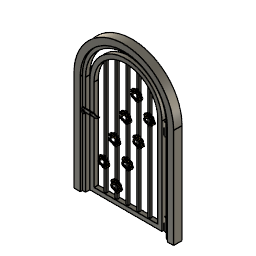
Dog+Door (Autodesk Fusion 360 archive; units mm, degrees)
design "Dog Door"
Autodesk Fusion 360 part; units mm, degrees
note: some values were not read from the file. Chosen so that the rebuilt part matches the saved one: which bodies a step acts on.
(part 1 of 3)
sketch "DJ - Baxley - Dog Door" plane through (0, 0, 0) normal (0, 1, 0) x (1, 0, 0)
  line L0 (607.7627, -514.9017) -> (801.2677, -514.9017)
  line L1 (607.7627, -512.0374) -> (758.5846, -512.0374)
  line L2 (418.6134, 33.8718) -> (522.0074, 33.8718)
  line L3 (418.6134, 36.7362) -> (541.7026, 36.7362)
  line L4 (-253.3508, 33.8718) -> (-95.7652, 33.8718)
  line L5 (-253.3508, 36.7362) -> (-129.8188, 36.7362)
  circle A0 centre (-152.9013, -288.0754) radius 7.1816
  circle A1 centre (-11.8765, -330.8233) radius 7.1816
  circle A2 centre (-21.6679, -658.9263) radius 7.1816
  circle A3 centre (53.7402, -526.3669) radius 7.1816
  circle A4 centre (-77.4932, -135.2797) radius 7.1816
  circle A5 centre (-87.2846, -473.5008) radius 7.1816
  arc A6 (65.6738, -526.867) -> (65.6738, -526.867) centre (53.7402, -526.3669) cw
  arc A7 (-9.7343, -659.4265) -> (-9.7343, -659.4265) centre (-21.6679, -658.9263) cw
  arc A8 (-140.9676, -288.5756) -> (-140.9676, -288.5756) centre (-152.9013, -288.0754) cw
  arc A9 (-65.5595, -135.7798) -> (-65.5595, -135.7798) centre (-77.4932, -135.2797) cw
  arc A10 (0.0572, -331.3234) -> (0.0572, -331.3234) centre (-11.8765, -330.8233) cw
  arc A11 (-75.351, -474.001) -> (-75.351, -474.001) centre (-87.2846, -473.5008) cw
  circle A12 centre (-61.241, -141.518) radius 7.1816
  circle A13 centre (69.9923, -532.6052) radius 7.1816
  circle A14 centre (-136.6492, -294.3137) radius 7.1816
  circle A15 centre (-71.0325, -479.7392) radius 7.1816
  circle A16 centre (4.3756, -337.0616) radius 7.1816
  circle A17 centre (-5.4158, -665.1646) radius 7.1816
  circle A18 centre (11.4514, -657.6558) radius 7.1816
  circle A19 centre (-44.3738, -134.0092) radius 7.1816
  circle A20 centre (21.2429, -329.5528) radius 7.1816
  circle A21 centre (-119.7819, -286.8049) radius 7.1816
  circle A22 centre (86.8596, -525.0964) radius 7.1816
  circle A23 centre (-54.1652, -472.2303) radius 7.1816
  arc A24 (-129.4885, -293.765) -> (-129.4885, -293.765) centre (-119.7819, -286.8049) cw
  arc A25 (1.7448, -664.6159) -> (1.7448, -664.6159) centre (11.4514, -657.6558) cw
  arc A26 (-54.0804, -140.9693) -> (-54.0804, -140.9693) centre (-44.3738, -134.0092) cw
  arc A27 (77.1529, -532.0565) -> (77.1529, -532.0565) centre (86.8596, -525.0964) cw
  arc A28 (-63.8719, -479.1905) -> (-63.8719, -479.1905) centre (-54.1652, -472.2303) cw
  arc A29 (11.5363, -336.5129) -> (11.5363, -336.5129) centre (21.2429, -329.5528) cw
  circle A30 centre (27.4799, -313.3013) radius 7.1825
  circle A31 centre (-47.9282, -455.9788) radius 7.1825
  circle A32 centre (-38.1368, -117.7577) radius 7.1825
  circle A33 centre (17.6884, -641.4043) radius 7.1825
  circle A34 centre (-113.5449, -270.5534) radius 7.1825
  circle A35 centre (93.0966, -508.8449) radius 7.1825
  arc A36 (-123.6388, -263.5828) -> (-125.432, -269.8418) centre (-116.4072, -269.0411) ccw
  arc A37 (61.7026, -517.6651) -> (60.8566, -516.7375) centre (51.8781, -525.7767) ccw
  arc A38 (81.2094, -508.1333) -> (81.353, -509.5872) centre (62.2283, -510.7421) cw
  arc A39 (-125.432, -269.8418) -> (-125.2884, -271.2957) centre (-144.4132, -272.4506) cw
  arc A40 (7.5945, -634.4337) -> (5.8013, -640.6927) centre (14.8261, -639.892) ccw
  arc A41 (-139.7053, -250.77) -> (-138.4238, -249.5216) centre (-127.7264, -261.7846) cw
  arc A42 (-75.2386, -123.1969) -> (-77.5786, -122.844) centre (-74.3062, -109.0815) cw
  arc A43 (54.9363, -493.7824) -> (58.1264, -493.5058) centre (54.4348, -469.4584) ccw
  arc A44 (-95.1258, -450.308) -> (-86.0885, -440.9163) centre (-84.8968, -451.1071) cw
  arc A45 (5.8013, -640.6927) -> (5.9449, -642.1466) centre (-13.1798, -643.3015) cw
  arc A46 (-59.8154, -455.2673) -> (-59.6718, -456.7212) centre (-78.7965, -457.8761) cw
  arc A47 (-50.0239, -117.0461) -> (-49.8803, -118.5) centre (-69.005, -119.6549) cw
  arc A48 (-72.8072, -434.947) -> (-58.0221, -449.0083) centre (-66.1625, -442.764) cw
  arc A49 (-59.6718, -456.7212) -> (-79.3222, -464.799) centre (-70.9412, -457.2469) cw
  arc A50 (45.899, -503.1741) -> (54.9363, -493.7824) centre (56.128, -503.9731) cw
  arc A51 (-152.9867, -275.6397) -> (-160.7425, -264.8826) centre (-150.5091, -265.6789) cw
  arc A52 (-150.6468, -275.9926) -> (-152.9867, -275.6397) centre (-149.7143, -261.8772) cw
  arc A53 (55.9947, -514.2841) -> (53.6548, -513.9312) centre (56.9271, -500.1687) cw
  arc A54 (-70.3768, -125.6503) -> (-75.2386, -123.1969) centre (-76.6948, -132.1266) ccw
  arc A55 (60.8566, -516.7375) -> (55.9947, -514.2841) centre (54.5386, -523.2138) ccw
  arc A56 (-64.2972, -97.9742) -> (-63.0157, -96.7259) centre (-52.3183, -108.9889) cw
  arc A57 (-73.107, -102.4186) -> (-64.2972, -97.9742) centre (-75.763, -86.2002) ccw
  arc A58 (-48.2307, -110.7871) -> (-50.0239, -117.0461) centre (-40.9991, -116.2454) ccw
  arc A59 (-77.5786, -122.844) -> (-85.3344, -112.0869) centre (-75.1009, -112.8832) cw
  arc A60 (-9.622, -318.7405) -> (-11.9619, -318.3876) centre (-8.6895, -304.6251) cw
  arc A61 (66.9361, -489.0615) -> (68.2176, -487.8131) centre (78.915, -500.0761) cw
  arc A62 (-7.4903, -297.9622) -> (1.3195, -293.5179) centre (-10.1463, -281.7438) ccw
  arc A63 (-3.9141, -322.1215) -> (-4.7601, -321.1939) centre (-13.7386, -330.2331) ccw
  arc A64 (-85.3344, -112.0869) -> (-76.297, -102.6952) centre (-75.1054, -112.8859) cw
  arc A65 (15.5928, -312.5897) -> (15.7364, -314.0436) centre (-3.3884, -315.1985) cw
  arc A66 (53.6548, -513.9312) -> (45.899, -503.1741) centre (56.1324, -503.9704) cw
  arc A67 (-82.8984, -440.6398) -> (-74.0887, -436.1954) centre (-85.5544, -424.4213) ccw
  arc A68 (58.1264, -493.5058) -> (66.9361, -489.0615) centre (55.4703, -477.2874) ccw
  arc A69 (-58.0221, -449.0083) -> (-59.8154, -455.2673) centre (-50.7905, -454.4665) ccw
  arc A70 (2.6009, -292.2695) -> (17.386, -306.3307) centre (9.2456, -300.0864) cw
  arc A71 (1.3195, -293.5179) -> (2.6009, -292.2695) centre (13.2983, -304.5325) cw
  arc A72 (-145.7849, -278.446) -> (-150.6468, -275.9926) centre (-152.1029, -284.9223) ccw
  arc A73 (-138.4238, -249.5216) -> (-123.6388, -263.5828) centre (-131.7791, -257.3385) cw
  arc A74 (-144.9389, -279.3736) -> (-145.7849, -278.446) centre (-154.7633, -287.4852) ccw
  arc A75 (-160.7425, -264.8826) -> (-151.7051, -255.4909) centre (-150.5135, -265.6816) cw
  arc A76 (-49.8803, -118.5) -> (-69.5307, -126.5778) centre (-61.1497, -119.0257) cw
  arc A77 (-69.5307, -126.5778) -> (-70.3768, -125.6503) centre (-79.3552, -134.6895) ccw
  arc A78 (-74.0887, -436.1954) -> (-72.8072, -434.947) centre (-62.1098, -447.2101) cw
  arc A79 (-7.1905, -620.3725) -> (7.5945, -634.4337) centre (-0.5458, -628.1894) cw
  arc A80 (-86.0885, -440.9163) -> (-82.8984, -440.6398) centre (-86.59, -416.5924) ccw
  arc A81 (-85.0301, -461.4181) -> (-87.37, -461.0652) centre (-84.0977, -447.3027) cw
  arc A82 (-4.7601, -321.1939) -> (-9.622, -318.7405) centre (-11.0781, -327.6702) ccw
  arc A83 (-87.37, -461.0652) -> (-95.1258, -450.308) centre (-84.8924, -451.1043) cw
  arc A84 (81.353, -509.5872) -> (61.7026, -517.6651) centre (70.0836, -510.1129) cw
  arc A85 (-79.3222, -464.799) -> (-80.1682, -463.8715) centre (-89.1467, -472.9106) ccw
  arc A86 (-125.2884, -271.2957) -> (-144.9389, -279.3736) centre (-136.5578, -271.8214) cw
  arc A87 (-76.297, -102.6952) -> (-73.107, -102.4186) centre (-76.7985, -78.3712) ccw
  arc A88 (83.0027, -501.8743) -> (81.2094, -508.1333) centre (90.2342, -507.3326) ccw
  arc A89 (-10.6804, -298.2388) -> (-7.4903, -297.9622) centre (-11.1819, -273.9148) ccw
  arc A90 (-151.7051, -255.4909) -> (-148.5151, -255.2144) centre (-152.2066, -231.1669) ccw
  arc A91 (-63.0157, -96.7259) -> (-48.2307, -110.7871) centre (-56.371, -104.5428) cw
  arc A92 (-13.7055, -650.2245) -> (-14.5516, -649.2969) centre (-23.53, -658.3361) ccw
  arc A93 (-80.1682, -463.8715) -> (-85.0301, -461.4181) centre (-86.4862, -470.3477) ccw
  arc A94 (-17.2817, -626.0653) -> (-8.472, -621.6209) centre (-19.9378, -609.8468) ccw
  arc A95 (-19.4134, -646.8435) -> (-21.7533, -646.4906) centre (-18.481, -632.7281) cw
  arc A96 (-11.9619, -318.3876) -> (-19.7177, -307.6305) centre (-9.4843, -308.4268) cw
  arc A97 (68.2176, -487.8131) -> (83.0027, -501.8743) centre (74.8623, -495.63) cw
  arc A98 (-148.5151, -255.2144) -> (-139.7053, -250.77) centre (-151.1711, -238.9959) ccw
  arc A99 (-29.5091, -635.7335) -> (-20.4718, -626.3418) centre (-19.2801, -636.5325) cw
  arc A100 (5.9449, -642.1466) -> (-13.7055, -650.2245) centre (-5.3245, -642.6723) cw
  arc A101 (15.7364, -314.0436) -> (-3.9141, -322.1215) centre (4.4669, -314.5693) cw
  arc A102 (-14.5516, -649.2969) -> (-19.4134, -646.8435) centre (-20.8696, -655.7732) ccw
  arc A103 (-8.472, -621.6209) -> (-7.1905, -620.3725) centre (3.5069, -632.6355) cw
  arc A104 (17.386, -306.3307) -> (15.5928, -312.5897) centre (24.6176, -311.789) ccw
  arc A105 (-19.7177, -307.6305) -> (-10.6804, -298.2388) centre (-9.4887, -308.4295) cw
  arc A106 (-20.4718, -626.3418) -> (-17.2817, -626.0653) centre (-20.9733, -602.0178) ccw
  arc A107 (-21.7533, -646.4906) -> (-29.5091, -635.7335) centre (-19.2757, -636.5298) cw
  arc A108 (-2.0837, -290.1836) -> (-0.5075, -288.6612) centre (13.2983, -304.5325) cw
  arc A109 (-77.4918, -432.8611) -> (-75.9156, -431.3388) centre (-62.1098, -447.2101) cw
  arc A110 (-10.9728, -293.4803) -> (-8.2372, -293.2586) centre (-11.1819, -273.9148) ccw
  arc A111 (-75.9156, -431.3388) -> (-51.2415, -444.5025) centre (-66.1625, -442.764) cw
  arc A112 (-34.2572, -635.3633) -> (-20.7643, -621.5833) centre (-19.2801, -636.5325) cw
  arc A113 (-6.6815, -341.5785) -> (-18.1828, -320.68) centre (-11.8765, -330.8234) cw
  arc A114 (-11.8752, -618.2866) -> (-10.2989, -616.7642) centre (3.5069, -632.6355) cw
  arc A115 (14.3752, -629.9279) -> (22.2071, -652.4617) centre (17.6884, -641.4043) cw
  arc A116 (-16.473, -669.6815) -> (-27.9743, -648.783) centre (-21.668, -658.9264) cw
  arc A117 (-93.591, -463.3575) -> (-99.8739, -449.9379) centre (-84.8924, -451.1043) cw
  arc A118 (81.5082, -535.7746) -> (58.9352, -537.1221) centre (69.9923, -532.6052) cw
  arc A119 (63.533, -485.7272) -> (65.1092, -484.2048) centre (78.915, -500.0761) cw
  arc A120 (47.4338, -516.2236) -> (41.1509, -502.8039) centre (56.1324, -503.9704) cw
  arc A121 (57.3795, -488.8022) -> (63.533, -485.7272) centre (55.4703, -477.2874) ccw
  arc A122 (41.1509, -502.8039) -> (54.6438, -489.0239) centre (56.128, -503.9731) cw
  arc A123 (89.7833, -497.3685) -> (97.6152, -519.9023) centre (93.0966, -508.8449) cw
  arc A124 (54.6438, -489.0239) -> (57.3795, -488.8022) centre (54.4348, -469.4584) ccw
  arc A125 (65.1092, -484.2048) -> (89.7833, -497.3685) centre (74.8623, -495.63) cw
  arc A126 (-66.1242, -93.1176) -> (-41.45, -106.2813) centre (-56.371, -104.5428) cw
  arc A127 (-86.3809, -436.1579) -> (-83.6453, -435.9362) centre (-86.59, -416.5924) ccw
  arc A128 (-143.1085, -247.4357) -> (-141.5323, -245.9133) centre (-127.7264, -261.7846) cw
  arc A129 (-159.2076, -277.9321) -> (-165.4906, -264.5124) centre (-150.5091, -265.6789) cw
  arc A130 (-49.7251, -144.6874) -> (-72.2982, -146.0349) centre (-61.241, -141.518) cw
  arc A131 (-141.5323, -245.9133) -> (-116.8581, -259.077) centre (-131.7791, -257.3385) cw
  arc A132 (-109.0263, -281.6108) -> (-125.1332, -297.4832) centre (-119.7819, -286.8049) cw
  arc A133 (-83.7995, -125.1364) -> (-90.0824, -111.7167) centre (-75.1009, -112.8832) cw
  arc A134 (-90.0824, -111.7167) -> (-76.5895, -97.9367) centre (-75.1054, -112.8859) cw
  arc A135 (-67.7004, -94.64) -> (-66.1242, -93.1176) centre (-52.3183, -108.9889) cw
  arc A136 (-165.4906, -264.5124) -> (-151.9976, -250.7324) centre (-150.5135, -265.6816) cw
  arc A137 (-76.5895, -97.9367) -> (-73.8539, -97.715) centre (-76.7985, -78.3712) ccw
  arc A138 (-125.1332, -297.4832) -> (-147.7063, -298.8306) centre (-136.6492, -294.3137) cw
  arc A139 (-82.0896, -484.2561) -> (-93.591, -463.3575) centre (-87.2847, -473.501) cw
  arc A140 (-116.8581, -259.077) -> (-109.0263, -281.6108) centre (-113.5449, -270.5534) cw
  arc A141 (-151.9976, -250.7324) -> (-149.262, -250.5107) centre (-152.2066, -231.1669) ccw
  arc A142 (-73.8539, -97.715) -> (-67.7004, -94.64) centre (-75.763, -86.2002) ccw
  arc A143 (-33.6181, -128.815) -> (-49.7251, -144.6874) centre (-44.3738, -134.0092) cw
  arc A144 (-72.2982, -146.0349) -> (-83.7995, -125.1364) centre (-77.4932, -135.2798) cw
  arc A145 (-147.7063, -298.8306) -> (-159.2076, -277.9321) centre (-152.9013, -288.0755) cw
  arc A146 (-149.262, -250.5107) -> (-143.1085, -247.4357) centre (-151.1711, -238.9959) ccw
  arc A147 (-41.45, -106.2813) -> (-33.6181, -128.815) centre (-38.1368, -117.7577) cw
  arc A148 (-99.8739, -449.9379) -> (-86.3809, -436.1579) centre (-84.8968, -451.1071) cw
  arc A149 (-43.4096, -467.0362) -> (-59.5166, -482.9086) centre (-54.1652, -472.2303) cw
  arc A150 (-8.2372, -293.2586) -> (-2.0837, -290.1836) centre (-10.1463, -281.7438) ccw
  arc A151 (-18.0287, -621.3616) -> (-11.8752, -618.2866) centre (-19.9378, -609.8468) ccw
  arc A152 (31.9985, -324.3586) -> (15.8916, -340.231) centre (21.2429, -329.5528) cw
  arc A153 (15.8916, -340.231) -> (-6.6815, -341.5785) centre (4.3756, -337.0616) cw
  arc A154 (97.6152, -519.9023) -> (81.5082, -535.7746) centre (86.8596, -525.0964) cw
  arc A155 (-18.1828, -320.68) -> (-24.4658, -307.2603) centre (-9.4843, -308.4268) cw
  arc A156 (-59.5166, -482.9086) -> (-82.0896, -484.2561) centre (-71.0325, -479.7392) cw
  arc A157 (-24.4658, -307.2603) -> (-10.9728, -293.4803) centre (-9.4887, -308.4295) cw
  arc A158 (-27.9743, -648.783) -> (-34.2572, -635.3633) centre (-19.2757, -636.5298) cw
  arc A159 (-83.6453, -435.9362) -> (-77.4918, -432.8611) centre (-85.5544, -424.4213) ccw
  arc A160 (-20.7643, -621.5833) -> (-18.0287, -621.3616) centre (-20.9733, -602.0178) ccw
  arc A161 (-0.5075, -288.6612) -> (24.1667, -301.8249) centre (9.2456, -300.0864) cw
  arc A162 (-51.2415, -444.5025) -> (-43.4096, -467.0362) centre (-47.9282, -455.9788) cw
  arc A163 (-10.2989, -616.7642) -> (14.3752, -629.9279) centre (-0.5458, -628.1894) cw
  arc A164 (22.2071, -652.4617) -> (6.1001, -668.3341) centre (11.4514, -657.6558) cw
  arc A165 (6.1001, -668.3341) -> (-16.473, -669.6815) centre (-5.4158, -665.1646) cw
  arc A166 (58.9352, -537.1221) -> (47.4338, -516.2236) centre (53.7401, -526.367) cw
  arc A167 (24.1667, -301.8249) -> (31.9985, -324.3586) centre (27.4799, -313.3013) cw
  line L6 (-608.6223, -1298.6439) -> (1173.7004, -1298.6439)
  line L7 (1173.7004, -1298.6439) -> (1173.7004, 250.0202)
  line L8 (1173.7004, 250.0202) -> (-608.6223, 250.0202)
  line L9 (-608.6223, 250.0202) -> (-608.6223, -1298.6439)
  line L10 (-241.1509, 0) -> (-241.1509, -411.8539)
  line L11 (241.4491, -596.9) -> (241.4491, 0)
  line L12 (-241.1509, -439.1647) -> (-241.1509, -596.9)
  arc A168 (-241.1509, -596.9) -> (241.4491, -596.9) centre (0.1491, -596.9) ccw
  line L13 (-215.7509, -439.1647) -> (-215.7509, -596.9)
  line L14 (-215.7509, -25.4) -> (-215.7509, -420.1147)
  line L15 (216.0491, -25.4) -> (-215.7509, -25.4)
  line L16 (216.0491, -596.9) -> (216.0491, -25.4)
  arc A169 (-215.7509, -596.9) -> (216.0491, -596.9) centre (0.1491, -596.9) ccw
  line L17 (-190.3509, -50.8) -> (-190.3509, -420.1147)
  arc A170 (-190.3509, -596.9) -> (190.6491, -596.9) centre (0.1491, -596.9) ccw
  line L18 (190.6491, -596.9) -> (190.6491, -50.8)
  line L19 (-190.3509, -439.1647) -> (-190.3509, -596.9)
  line L20 (190.6491, -50.8) -> (-190.3509, -50.8)
  circle A171 centre (-203.0509, -429.6397) radius 6.35
  line L21 (-253.8509, -411.8539) -> (-241.1509, -411.8539)
  line L22 (-241.1509, -411.8539) -> (-241.1509, -428.0522)
  line L23 (-253.8509, -428.0522) -> (-253.8509, -411.8539)
  line L24 (-241.1509, -428.0522) -> (-253.8509, -428.0522)
  line L25 (-181.8374, -420.1147) -> (-241.1509, -420.1147)
  line L26 (-255.4225, -439.1647) -> (-186.7302, -439.1647)
  arc A172 (-184.4429, -438.341) -> (-152.1305, -436.5446) centre (-167.2009, -456.9736) cw
  line L27 (-253.8509, -420.1147) -> (-255.4225, -420.1147)
  arc A173 (-152.1305, -436.5446) -> (-151.004, -435.1368) centre (-151.705, -435.7305) ccw
  arc A174 (-151.004, -435.1368) -> (-181.8374, -420.1147) centre (-180.7971, -457.1339) ccw
  arc A175 (-255.4225, -420.1147) -> (-255.4225, -439.1647) centre (-230.008, -429.6397) ccw
  arc A176 (-186.7302, -439.1647) -> (-184.4429, -438.341) centre (-186.7379, -435.5556) ccw
  line L28 (222.3991, -25.4) -> (235.0991, -25.4)
  line L29 (222.3991, -101.6) -> (222.3991, -25.4)
  line L30 (235.0991, -25.4) -> (235.0991, -101.6)
  line L31 (235.0991, -101.6) -> (222.3991, -101.6)
  line L32 (222.3991, -63.5) -> (235.0991, -63.5)
  line L33 (222.3991, -25.4) -> (216.0491, -25.4)
  line L34 (222.3991, -63.5) -> (222.3991, -25.4)
  line L35 (216.0491, -63.5) -> (222.3991, -63.5)
  line L36 (216.0491, -25.4) -> (216.0491, -63.5)
  line L37 (235.0991, -101.6) -> (241.4491, -101.6)
  line L38 (241.4491, -101.6) -> (241.4491, -63.5)
  line L39 (241.4491, -63.5) -> (235.0991, -63.5)
  line L40 (235.0991, -63.5) -> (235.0991, -101.6)
  line L41 (222.3991, -594.9254) -> (222.3991, -518.7254)
  line L42 (235.0991, -518.7254) -> (235.0991, -594.9254)
  line L43 (222.3991, -518.7254) -> (235.0991, -518.7254)
  line L44 (235.0991, -594.9254) -> (222.3991, -594.9254)
  line L45 (222.3991, -556.8254) -> (235.0991, -556.8254)
  line L46 (222.3991, -556.8254) -> (222.3991, -518.7254)
  line L47 (216.0491, -518.7254) -> (216.0491, -556.8254)
  line L48 (216.0491, -556.8254) -> (222.3991, -556.8254)
  line L49 (222.3991, -518.7254) -> (216.0491, -518.7254)
  line L50 (235.0991, -594.9254) -> (241.4491, -594.9254)
  line L51 (241.4491, -556.8254) -> (235.0991, -556.8254)
  line L52 (241.4491, -594.9254) -> (241.4491, -556.8254)
  line L53 (235.0991, -556.8254) -> (235.0991, -594.9254)
  line L54 (6.4991, -50.8) -> (6.4991, -285.3177)
  line L55 (6.4991, -290.2014) -> (6.4991, -325.6665)
  line L56 (6.4991, -330.2011) -> (6.4991, -343.9221)
  line L57 (6.4991, -348.8155) -> (6.4991, -614.9219)
  line L58 (6.4991, -620.7312) -> (6.4991, -636.3213)
  line L59 (6.4991, -652.4548) -> (6.4991, -662.8568)
  line L60 (6.4991, -668.5249) -> (6.4991, -787.2941)
  line L61 (-6.2009, -50.8) -> (-6.2009, -292.7287)
  line L62 (-6.2009, -297.6977) -> (-6.2009, -320.3138)
  line L63 (-6.2009, -326.4229) -> (-6.2009, -335.2236)
  line L64 (-6.2009, -342.6114) -> (-6.2009, -614.2725)
  line L65 (-6.2009, -619.6292) -> (-6.2009, -653.9199)
  line L66 (-6.2009, -658.0261) -> (-6.2009, -672.3032)
  line L67 (-6.2009, -677.083) -> (-6.2009, -787.2941)
  line L68 (-59.1175, -50.8) -> (-59.1175, -89.7741)
  line L69 (-59.1175, -94.6578) -> (-59.1175, -130.1228)
  line L70 (-59.1175, -134.6575) -> (-59.1175, -148.3785)
  line L71 (-59.1175, -153.2719) -> (-59.1175, -429.4964)
  line L72 (-59.1175, -435.3057) -> (-59.1175, -450.8958)
  line L73 (-59.1175, -467.0293) -> (-59.1175, -477.4313)
  line L74 (-59.1175, -483.0994) -> (-59.1175, -777.9462)
  line L75 (-71.8175, -50.8) -> (-71.8175, -97.1851)
  line L76 (-71.8175, -102.1541) -> (-71.8175, -124.5061)
  line L77 (-71.8175, -130.8793) -> (-71.8175, -139.68)
  line L78 (-71.8175, -147.0678) -> (-71.8175, -428.8471)
  line L79 (-71.8175, -434.2038) -> (-71.8175, -468.4945)
  line L80 (-71.8175, -472.6006) -> (-71.8175, -486.8778)
  line L81 (-71.8175, -491.6575) -> (-71.8175, -773.2832)
  line L82 (72.1158, -50.8) -> (72.1158, -480.8613)
  line L83 (72.1158, -485.745) -> (72.1158, -521.2101)
  line L84 (72.1158, -525.7447) -> (72.1158, -539.4657)
  line L85 (72.1158, -544.3591) -> (72.1158, -773.2832)
  line L86 (59.4158, -50.8) -> (59.4158, -488.2723)
  line L87 (59.4158, -493.2413) -> (59.4158, -515.8574)
  line L88 (59.4158, -521.9665) -> (59.4158, -530.7672)
  line L89 (59.4158, -538.155) -> (59.4158, -777.9462)
  line L90 (137.7325, -50.8) -> (137.7325, -728.6614)
  line L91 (125.0325, -50.8) -> (125.0325, -740.7555)
  line L92 (-124.7342, -50.8) -> (-124.7342, -244.071)
  line L93 (-124.7342, -249.8803) -> (-124.7342, -265.4704)
  line L94 (-124.7342, -281.6039) -> (-124.7342, -292.0059)
  line L95 (-124.7342, -297.674) -> (-124.7342, -740.7555)
  line L96 (-137.4342, -50.8) -> (-137.4342, -243.4216)
  line L97 (-137.4342, -248.7783) -> (-137.4342, -283.069)
  line L98 (-137.4342, -287.1751) -> (-137.4342, -301.4523)
  line L99 (-137.4342, -285.9415) -> (-137.4342, -728.6614)
  line L100 (460.8307, -38.1) -> (486.2307, -38.1)
  line L101 (460.8307, -12.7) -> (460.8307, -38.1)
  line L102 (486.2307, -12.7) -> (460.8307, -12.7)
  line L103 (486.2307, -38.1) -> (486.2307, -12.7)
  line L104 (943.4307, -12.7) -> (511.6307, -12.7)
  line L105 (943.4307, -38.1) -> (943.4307, -12.7)
  line L106 (511.6307, -12.7) -> (511.6307, -38.1)
  line L107 (511.6307, -38.1) -> (943.4307, -38.1)
  line L108 (517.9807, -12.7) -> (517.9807, -9.356)
  line L109 (530.6807, -12.7) -> (530.6807, -9.356)
  line L110 (473.5307, -12.7) -> (473.5307, -9.356)
  line L111 (486.2307, -12.7) -> (486.2307, -9.356)
  line L112 (540.5255, -9.356) -> (469.714, -9.356)
  line L113 (469.714, -6.181) -> (540.5255, -6.181)
  line L114 (540.5255, -6.181) -> (540.5255, -9.356)
  line L115 (469.714, -9.356) -> (469.714, -6.181)
  line L116 (473.5307, -6.181) -> (473.5307, -2.837)
  line L117 (486.2307, -6.181) -> (486.2307, -2.837)
  line L118 (473.5307, -2.837) -> (486.2307, -2.837)
  line L119 (994.2307, -38.1) -> (994.2307, -12.7)
  line L120 (994.2307, -12.7) -> (968.8307, -12.7)
  line L121 (968.8307, -12.7) -> (968.8307, -38.1)
  line L122 (968.8307, -38.1) -> (994.2307, -38.1)
  line L123 (962.4807, -12.7) -> (962.4807, -38.1)
  line L124 (968.8307, -38.1) -> (968.8307, -12.7)
  line L125 (968.8307, -12.7) -> (962.4807, -12.7)
  line L126 (962.4807, -38.1) -> (968.8307, -38.1)
  line L127 (949.7807, -38.1) -> (949.7807, -12.7)
  line L128 (943.4307, -38.1) -> (949.7807, -38.1)
  line L129 (949.7807, -12.7) -> (943.4307, -12.7)
  line L130 (943.4307, -12.7) -> (943.4307, -38.1)
  circle A177 centre (956.1307, -12.7) radius 6.35
  arc A178 (260.4991, -596.9) -> (-260.2009, -596.9) centre (0.1491, -596.9) cw
  line L131 (260.4991, 0) -> (260.4991, -596.9)
  line L132 (-260.2009, -596.9) -> (-260.2009, 0)
  line L133 (460.8307, -12.7) -> (467.1807, -12.7)
  line L134 (467.1807, -7.9375) -> (429.0807, -7.9375)
  line L135 (467.1807, -12.7) -> (467.1807, -7.9375)
  line L136 (429.0807, -7.9375) -> (429.0807, -12.7)
  line L137 (1026.0501, -7.9375) -> (1026.0501, -12.7)
  line L138 (987.9501, -12.7) -> (987.9501, -7.9375)
  line L139 (987.9501, -7.9375) -> (1026.0501, -7.9375)
  line L140 (467.1807, -189.5481) -> (987.9501, -189.5481)
  line L141 (-298.3009, -596.9) -> (-298.3009, 0)
  arc A179 (298.5991, -596.9) -> (-298.3009, -596.9) centre (0.1491, -596.9) cw
  line L142 (298.5991, 0) -> (298.5991, -596.9)
  circle A180 centre (654.6615, -728.3062) radius 28.7265
  arc A181 (702.3961, -730.3068) -> (702.3961, -730.3068) centre (654.6615, -728.3062) cw
  circle A182 centre (719.6699, -753.2596) radius 28.7265
  circle A183 centre (787.139, -723.2242) radius 28.7265
  arc A184 (748.3124, -751.0647) -> (748.3124, -751.0647) centre (787.139, -723.2242) cw
  circle A185 centre (812.087, -658.2181) radius 28.7301
  arc A186 (707.4452, -579.0845) -> (712.5712, -574.091) centre (755.3608, -623.1431) cw
  arc A187 (771.7114, -630.3359) -> (764.5384, -655.372) centre (800.6377, -652.169) ccw
  arc A188 (659.446, -597.9682) -> (672.2062, -596.862) centre (657.44, -500.6724) ccw
  arc A189 (654.3198, -678.5635) -> (623.2966, -635.535) centre (664.2303, -638.7201) cw
  arc A190 (623.2966, -635.535) -> (659.446, -597.9682) centre (664.2126, -638.731) cw
  arc A191 (663.6795, -679.9752) -> (654.3198, -678.5635) centre (667.4092, -623.5135) cw
  arc A192 (712.5712, -574.091) -> (771.7114, -630.3359) centre (739.15, -605.3587) cw
  arc A193 (672.2062, -596.862) -> (707.4452, -579.0845) centre (661.5821, -531.9882) ccw
  arc A194 (764.5384, -655.372) -> (765.1128, -661.1875) centre (688.6139, -665.8071) cw
  arc A195 (765.1128, -661.1875) -> (686.5111, -693.4989) centre (720.0352, -663.2904) cw
  arc A196 (683.1269, -689.7887) -> (663.6795, -679.9752) centre (657.855, -715.6938) ccw
  arc A197 (686.5111, -693.4989) -> (683.1269, -689.7887) centre (647.2131, -725.9453) ccw
  arc A198 (675.4413, -771.3271) -> (629.436, -687.7329) centre (654.6613, -728.3068) cw
  arc A199 (669.2186, -578.0475) -> (693.8326, -565.7473) centre (661.5821, -531.9882) ccw
  arc A200 (629.436, -687.7329) -> (604.3043, -634.0543) centre (664.2303, -638.7201) cw
  arc A201 (693.8326, -565.7473) -> (700.1374, -559.6579) centre (755.3608, -623.1431) cw
  arc A202 (604.3043, -634.0543) -> (658.2761, -578.9344) centre (664.2126, -638.731) cw
  arc A203 (658.2761, -578.9344) -> (669.2186, -578.0475) centre (657.44, -500.6724) ccw
  arc A204 (765.7337, -765.9373) -> (675.4413, -771.3271) centre (719.6699, -753.2596) cw
  arc A205 (830.1615, -702.4477) -> (765.7337, -765.9373) centre (787.139, -723.2242) cw
  arc A206 (798.834, -612.3128) -> (830.1615, -702.4477) centre (812.087, -658.2181) cw
  arc A207 (700.1374, -559.6579) -> (798.834, -612.3128) centre (739.15, -605.3587) cw
  arc A208 (884.2022, -372.9919) -> (903.2522, -353.9419) centre (903.2522, -372.9919) cw
  line L143 (541.3022, -372.9919) -> (884.2022, -372.9919)
  arc A209 (560.3522, -220.5919) -> (541.3022, -239.6419) centre (541.3022, -220.5919) cw
  line L144 (903.2522, -353.9419) -> (903.2522, -220.5919)
  line L145 (903.2522, -220.5919) -> (560.3522, -220.5919)
  line L146 (541.3022, -239.6419) -> (541.3022, -372.9919)
  line L147 (912.7772, -211.0669) -> (912.7772, -382.5169)
  line L148 (912.7772, -211.0669) -> (531.7772, -211.0669)
  line L149 (531.7772, -211.0669) -> (531.7772, -382.5169)
  line L150 (531.7772, -382.5169) -> (912.7772, -382.5169)
  line L151 (320.6208, 0) -> (-320.6208, 0)
  line L152 (403.6807, -26.9875) -> (403.6807, -115.8875)
  line L153 (365.5807, -115.8875) -> (365.5807, -26.9875)
  line L154 (365.5807, -26.9875) -> (403.6807, -26.9875)
  line L155 (1089.5501, -115.8875) -> (1089.5501, -26.9875)
  line L156 (403.6807, -115.8875) -> (365.5807, -115.8875)
  line L157 (1051.4501, -115.8875) -> (1089.5501, -115.8875)
  line L158 (1051.4501, -26.9875) -> (1051.4501, -115.8875)
  line L159 (1089.5501, -26.9875) -> (1051.4501, -26.9875)
  line L160 (1089.5501, -26.9875) -> (1051.4501, -115.8875)
  line L161 (365.5807, -26.9875) -> (403.6807, -115.8875)
  line L162 (1051.4501, -26.9875) -> (1089.5501, -115.8875)
  line L163 (403.6807, -26.9875) -> (365.5807, -115.8875)
  line L164 (1013.3501, -115.8875) -> (1013.3501, -26.9875)
  line L165 (1106.7139, -115.8875) -> (1013.3501, -115.8875)
  line L166 (1013.3501, -26.9875) -> (1106.7139, -26.9875)
  line L167 (1013.3501, -26.9875) -> (1051.4501, -115.8875)
  line L168 (1051.4501, -26.9875) -> (1013.3501, -115.8875)
  line L169 (1051.4501, -115.8875) -> (1051.4501, -26.9875)
  line L170 (348.4169, -115.8875) -> (441.7807, -115.8875)
  line L171 (441.7807, -26.9875) -> (348.4169, -26.9875)
  line L172 (441.7807, -115.8875) -> (441.7807, -26.9875)
  line L173 (441.7807, -26.9875) -> (403.6807, -115.8875)
  line L174 (403.6807, -26.9875) -> (441.7807, -115.8875)
  line L175 (403.6807, -115.8875) -> (403.6807, -26.9875)
  line L176 (994.3001, -149.225) -> (1013.3501, -12.7)
  line L177 (994.3001, -12.7) -> (1013.3501, -149.225)
  line L178 (1013.3501, -149.225) -> (994.3001, -149.225)
  line L179 (994.3001, -149.225) -> (994.3001, -12.7)
  line L180 (994.3001, -12.7) -> (1013.3501, -12.7)
  line L181 (1013.3501, -12.7) -> (1013.3501, -149.225)
  line L182 (460.8307, -149.225) -> (441.7807, -12.7)
  line L183 (460.8307, -12.7) -> (441.7807, -149.225)
  line L184 (460.8307, -12.7) -> (441.7807, -12.7)
  line L185 (460.8307, -149.225) -> (460.8307, -12.7)
  line L186 (441.7807, -12.7) -> (441.7807, -149.225)
  line L187 (441.7807, -149.225) -> (460.8307, -149.225)
  line L188 (352.4174, -149.225) -> (441.7807, -130.175)
  line L189 (441.7807, -149.225) -> (352.4174, -130.175)
  line L190 (441.7807, -149.225) -> (441.7807, -130.175)
  line L191 (352.4174, -130.175) -> (352.4174, -149.225)
  line L192 (441.7807, -130.175) -> (352.4174, -130.175)
  line L193 (352.4174, -149.225) -> (441.7807, -149.225)
  line L194 (1102.7134, -149.225) -> (1013.3501, -130.175)
  line L195 (1013.3501, -149.225) -> (1102.7134, -130.175)
  line L196 (1102.7134, -130.175) -> (1102.7134, -149.225)
  line L197 (1013.3501, -130.175) -> (1102.7134, -130.175)
  line L198 (1102.7134, -149.225) -> (1013.3501, -149.225)
  line L199 (1013.3501, -149.225) -> (1013.3501, -130.175)
  line L200 (1112.4796, -12.7) -> (994.3001, -12.7)
  line L201 (1013.3501, -130.175) -> (1112.4796, -130.175)
  line L202 (342.6512, -12.7) -> (460.8307, -12.7)
  line L203 (441.7807, -130.175) -> (342.6512, -130.175)
  line L204 (-241.1509, -428.0522) -> (-241.1509, -439.1647)
  line L205 (-215.7509, -420.1147) -> (-215.7509, -439.1647)
  line L206 (-190.3509, -439.1647) -> (-190.3509, -420.1147)
  constraint perpendicular L26 L204
  constraint perpendicular L26 L205
  constraint perpendicular L25 L206
sketch "Sketch2" plane through (0, 0, 0) normal (0, 1, 0) x (1, 0, 0)
  line L0 (317.5, 0) -> (-317.5, 0)
  line L1 (-260.2009, -596.9) -> (-260.2009, 0)
  dimension "d1" = 635
  constraint midpoint origin L0
  constraint horizontal L0
  constraint vertical L1
  measures "d1" distance of L0.end L0.start
extrude "Extrude1" add sketch "DJ - Baxley - Dog Door" along normal mid plane 50.8 contours A178 L131 L132 L141 A179 L142 L151 makes body 1
extrude "Extrude2" add sketch "DJ - Baxley - Dog Door" along normal mid plane 25.4 separate body contours L10 L11 L12 A168 L21 L23 L26 L27 A175 L38 L52 A178 L131 L132 L151 | L23 L24 L26 L27 A175 L204 | L21 L22 L23 L24 makes body 2
extrude "Extrude3" add sketch "DJ - Baxley - Dog Door" along normal mid plane 25.4 separate body contours L13 L14 L15 L16 A169 L17 A170 L18 L19 L20 L25 L26 L36 L47 | L25 L26 L205 L206 | A171 makes body 3
sketch "Sketch3" plane through (0, 0, 0) normal (0, 1, 0) x (1, 0, 0)
  line L0 (-124.7342, -50.8) -> (-124.7342, -244.071)
  line L1 (-137.4342, -50.8) -> (-137.4342, -243.4216)
  line L2 (-124.7342, -297.674) -> (-124.7342, -740.7555)
  line L3 (-137.4342, -285.9415) -> (-137.4342, -728.6614)
  line L4 (-71.8175, -50.8) -> (-71.8175, -97.1851)
  line L5 (-59.1175, -50.8) -> (-59.1175, -89.7741)
  line L6 (-71.8175, -491.6575) -> (-71.8175, -773.2832)
  line L7 (-59.1175, -483.0994) -> (-59.1175, -777.9462)
  line L8 (-6.2009, -677.083) -> (-6.2009, -787.2941)
  line L9 (6.4991, -668.5249) -> (6.4991, -787.2941)
  line L10 (-6.2009, -50.8) -> (-6.2009, -292.7287)
  line L11 (6.4991, -50.8) -> (6.4991, -285.3177)
  line L12 (59.4158, -50.8) -> (59.4158, -488.2723)
  line L13 (72.1158, -50.8) -> (72.1158, -480.8613)
  line L14 (59.4158, -538.155) -> (59.4158, -777.9462)
  line L15 (72.1158, -544.3591) -> (72.1158, -773.2832)
  line L16 (125.0325, -50.8) -> (125.0325, -740.7555)
  line L17 (137.7325, -50.8) -> (137.7325, -728.6614)
  line L18 (-137.4342, -50.8) -> (-137.4342, -728.6614)
  line L19 (-124.7342, -740.7555) -> (-124.7342, -50.8)
  arc A0 (-190.3509, -596.9) -> (190.6491, -596.9) centre (0.1491, -596.9) ccw
  line L20 (190.6491, -596.9) -> (190.6491, -50.8)
  line L21 (190.6491, -50.8) -> (-190.3509, -50.8)
  line L22 (-190.3509, -50.8) -> (-190.3509, -596.9)
  line L23 (-215.7509, -25.4) -> (216.0491, -25.4)
  line L24 (216.0491, -25.4) -> (216.0491, -596.9)
  arc A1 (-215.7509, -596.9) -> (216.0491, -596.9) centre (0.1491, -596.9) ccw
  line L25 (-215.7509, -596.9) -> (-215.7509, -25.4)
  line L26 (-71.8175, -773.2832) -> (-71.8175, -50.8)
  line L27 (-59.1175, -50.8) -> (-59.1175, -777.9462)
  line L28 (-6.2009, -50.8) -> (-6.2009, -787.2941)
  line L29 (6.4991, -787.2941) -> (6.4991, -50.8)
  line L30 (59.4158, -50.8) -> (59.4158, -777.9462)
  line L31 (72.1158, -773.2832) -> (72.1158, -50.8)
  line L32 (125.0325, -50.8) -> (125.0325, -740.7555)
  line L33 (137.7325, -728.6614) -> (137.7325, -50.8)
  constraint coincident L1.start L18.start
  constraint coincident L3.end L18.end
  constraint coincident L2.end L19.start
  constraint coincident L0.start L19.end
  constraint coincident L6.end L26.start
  constraint coincident L4.start L26.end
  constraint coincident L5.start L27.start
  constraint coincident L7.end L27.end
  constraint coincident L10.start L28.start
  constraint coincident L8.end L28.end
  constraint coincident L9.end L29.start
  constraint coincident L11.start L29.end
  constraint coincident L12.start L30.start
  constraint coincident L14.end L30.end
  constraint coincident L15.end L31.start
  constraint coincident L13.start L31.end
  constraint coincident L16.start L32.start
  constraint coincident L16.end L32.end
  constraint coincident L17.end L33.start
  constraint coincident L17.start L33.end
extrude "Extrude4" add sketch "Sketch3" along normal mid plane 12.7 contours L0 L1 L2 L3 L18 L19 A0 L21 | L4 L5 L6 L7 A0 L21 L26 L27 | L8 L9 L10 L11 A0 L21 L28 L29 | L12 L13 L14 L15 A0 L21 L30 L31 | L16 L17 A0 L21 L32 L33 bodies 3